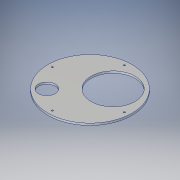
# Autodesk Inventor part: mini 55K stage
Saved by Autodesk Inventor 2018 (Build 220112000, 112)
## iProperties
Created: 2018-10-16
Part Number: mini 55K stage
Material: Aluminum 6061
Document SubType Name: Modeling
Designer: freyja
Density: 2.7 g/cm^3
Appearance: Aluminum - Flat
Mass: 655.353 g
Surface Area: 860.17 cm^2
Volume: 242.723 cm^3
Author: freyja
Autodesk Inventor part; units mm, degrees
ref_plane "YZ Plane" through (0, 0, 0) normal (1, 0, 0) x (0, 1, 0)
ref_plane "XZ Plane" through (0, 0, 0) normal (0, 1, 0) x (-1, 0, 0)
ref_plane "XY Plane" through (0, 0, 0) normal (0, 0, 1) x (1, 0, 0)
sketch "Sketch2" plane through (0, 0, 0) normal (0, 1, 0) x (-1, 0, 0)
  line L0 (0, 0) -> (-28.0184, -28.0184) construction
  line L1 (0, 0) -> (-39.624, 0) construction
  circle A0 centre (-28.0184, -28.0184) radius 133.35
  dimension "d6" = 39.624
  dimension "d7" = 315
  dimension "d8" = 266.7
  constraints: 4 end point, 1 centre point, 1 coincident, 1 equal length, 1 horizontal
  measures "d6" distance of L0.start L0.end
  measures "d8" diameter of A0
extrude "Extrusion1" add sketch "Sketch2" against normal blind 6.35
sketch "Sketch1" plane through (0, 0, 0) normal (0, 1, 0) x (-1, 0, 0)
  line L0 (0, 0) -> (-64.6578, -64.6578) construction
  line L1 (0, 0) -> (91.44, 0) construction
  circle A0 centre (-64.6578, -64.6578) radius 69.85
  line L2 (0, 0) -> (40.4112, 40.4112) construction
  line L3 (0, 0) -> (57.15, 0) construction
  circle A1 centre (40.4112, 40.4112) radius 26.67
  dimension "d0" = 91.44
  dimension "d1" = 135
  dimension "d2" = 139.7
  dimension "d3" = 57.15
  dimension "d4" = 45
  dimension "d5" = 53.34
  constraints: 8 end point, 2 centre point, 2 coincident, 2 equal length, 2 horizontal
  measures "d0" distance of L0.start L0.end
  measures "d1" angle of L0 L1
  measures "d2" diameter of A0
  measures "d3" distance of L0.start L2.end
  measures "d4" angle of L3 L2
  measures "d5" diameter of A1
extrude "Extrusion2" cut sketch "Sketch1" against normal up to surface (6.35 mm away)
sketch "Sketch5" plane through (0, 0, 0) normal (0, 1, 0) x (-1, 0, 0)
  line L0 (0, 0) -> (0, -165.1) construction
  line L1 (0, 0) -> (165.1, 0) construction
  line L2 (0, -165.1) -> (-17.9605, -147.1395)
  line L3 (0, 0) -> (-165.1, 0) construction
  line L4 (0, 0) -> (165.1, 0) construction
  line L5 (-165.1, 0) -> (-147.1395, -17.9605)
  line L6 (0, 0) -> (-28.0184, -28.0184) construction
  line L7 (0, 0) -> (39.624, 0) construction
  line L8 (-28.0184, -28.0184) -> (91.514, -28.0184)
  line L9 (-28.0184, -28.0184) -> (91.514, -28.0184) construction
  line L10 (-28.0184, -28.0184) -> (-28.0184, 91.514)
  line L11 (-28.0184, -28.0184) -> (91.514, -28.0184) construction
  dimension "d44" = 165.1
  dimension "d45" = 90
  dimension "d46" = 25.4
  dimension "d47" = 45
  dimension "d48" = 165.1
  dimension "d49" = 180
  dimension "d50" = 25.4
  dimension "d51" = 45
  dimension "d52" = 39.624
  dimension "d53" = 135
  dimension "d54" = 119.5324
  dimension "d55" = 0
  dimension "d56" = 119.5324
  dimension "d57" = 90
  constraints: 24 end point, 6 horizontal, 5 equal length, 2 vertical, 1 perpendicular
  measures "d44" distance of L0.start L0.end
  measures "d45" angle of L0 L1
  measures "d46" distance of L0.end L2.end
  measures "d47" angle of L0 L2
  measures "d48" distance of L0.start L3.end
  measures "d49" angle of L3 L4
  measures "d50" distance of L3.end L5.end
  measures "d51" angle of L5 L3
  measures "d52" distance of L0.start L6.end
  measures "d53" angle of L6 L7
  measures "d54" distance of L6.end L8.end
  measures "d55" distance between parallel lines of L8 L9
  measures "d56" distance of L6.end L10.end
  measures "d57" angle of L11 L10
hole "Hole2" at (28.0184, 0, 91.514) at (-91.514, 0, -28.0184) at (17.9605, 0, -147.1395) at (147.1395, 0, -17.9605) direction (0, -1, 0) diameter 4.9784 end through all thread size "1/4-20 UNC" class "2B" standard "ANSI Unified Screw Threads"
body "Solid1"
